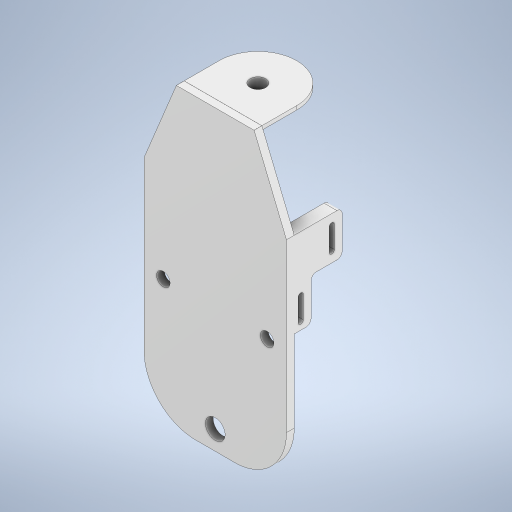
# Autodesk Inventor part: Electromagnet Gantry Plate
Saved by Autodesk Inventor 2023.2 (Build 272271030, 271C)
## iProperties
Created: 2023-04-10
Part Number: Electromagnet Gantry Plate
Material: PC/ABS Plastic
Document SubType Name: Modeling
Designer: ethan
Density: 0.357273 g/cm^3
Appearance: Smooth - White
Author: ethan
Autodesk Inventor part; units mm, degrees
ref_plane "YZ Plane" through (0, 0, 0) normal (1, 0, 0) x (0, 1, 0)
ref_plane "XZ Plane" through (0, 0, 0) normal (0, 1, 0) x (-1, 0, 0)
ref_plane "XY Plane" through (0, 0, 0) normal (0, 0, 1) x (1, 0, 0)
sketch "Sketch1" plane through (0, 0, 0) normal (0, 1, 0) x (-1, 0, 0)
  line L0 (0, 0) -> (55, 0)
  line L1 (55, 0) -> (55, -55)
  line L2 (55, -55) -> (0, -55)
  line L3 (0, -55) -> (0, 0)
  line L4 (47.55, -7.45) -> (7.45, -7.45) construction
  line L5 (7.45, -7.45) -> (7.45, -47.55) construction
  line L6 (7.45, -47.55) -> (47.55, -47.55) construction
  line L7 (47.55, -47.55) -> (47.55, -7.45) construction
  circle A0 centre (47.55, -7.45) radius 2.6
  circle A1 centre (47.55, -47.55) radius 2.6
  circle A2 centre (7.45, -47.55) radius 2.6
  circle A3 centre (7.45, -7.45) radius 2.6
  circle A4 centre (47.55, -7.45) radius 12.5 construction
  circle A5 centre (27.5, -7.45) radius 3.8
  line L8 (55, -55) -> (0, -55)
  line L9 (0, -55) -> (0, -139.9)
  line L10 (0, -139.9) -> (55, -139.9)
  line L11 (55, -139.9) -> (55, -55)
  point P0 (3.72, -55)
  dimension "d0" = 55
  dimension "d1" = 55
  dimension "d2" = 40.1
  dimension "d3" = 40.1
  dimension "d4" = 5.2
  dimension "d5" = 5.2
  dimension "d6" = 5.2
  dimension "d7" = 5.2
  dimension "d8" = 7.45
  dimension "d9" = 7.45
  dimension "d13" = 25
  dimension "d78" = 7.6
  dimension "d160" = 84.9
  constraints: 24 end point, 6 centre point, 6 parallel, 5 coincident, 3 horizontal, 3 perpendicular, 1 midpoint
  measures "d0" distance of L1.end L2.end
  measures "d1" distance of L0.end L1.end
  measures "d2" distance of L6.end L5.end
  measures "d3" distance of L5.end L4.end
  measures "d4" diameter of A0
  measures "d5" diameter of A3
  measures "d6" diameter of A1
  measures "d7" diameter of A2
  measures "d8" distance between parallel lines of L1 L7
  measures "d9" distance from line of L2 L5.end
  measures "d13" diameter of A4
  measures "d78" diameter of A5
  measures "d160" distance of L2.end L9.end
extrude "Extrusion1" add sketch "Sketch1" along normal blind 3 contours L0 L1 L2 L3 | L2 L11 L10 L9 | A0 | A3
fillet "Fillet1" radius 20 2 edges at (-55, 1.5, 0) (0, 1.5, 0)
ref_plane "Work Plane14" through (0, 0, 0) normal (0, 1, 0) x (1, 0, 0)
sketch "Sketch7" plane through (0, 0, 0) normal (0, 1, 0) x (1, 0, 0)
  line L0 (-19.45, 63) -> (-19.45, 55)
  line L1 (-35.55, 19.45) -> (-35.55, 63) projected
  line L2 (-19.45, 55) -> (-35.55, 55)
  line L3 (-35.55, 55) -> (-35.55, 63)
  line L4 (-35.55, 63) -> (-19.45, 63)
  line L5 (-19.45, 63) -> (-19.45, 55)
  circle A0 centre (-47.55, 47.55) radius 2.6 projected
  circle A1 centre (-47.55, 47.55) radius 12
  circle A2 centre (-7.45, 47.55) radius 2.6 projected
  circle A3 centre (-7.45, 47.55) radius 12
  point P0 (0, 0)
  point P1 (-53, 55)
  dimension "d67" = 24
  dimension "d68" = 24
  constraints: 10 end point, 2 centre point, 2 coincident, 2 parallel, 1 horizontal, 1 perpendicular
  measures "d67" diameter of A1
  measures "d68" diameter of A3
extrude "Extrusion9" add sketch "Sketch7" along normal blind 25 contours L0 L2 L1 L4
ref_plane "Work Plane2" through (-19.45, -5, -63) normal (0, 0, -1) x (-1, 0, 0)
sketch "Sketch9" plane through (-19.45, -5, -63) normal (0, 0, -1) x (-1, 0, 0)
  line L0 (0, 0) -> (0, 8) projected
  line L1 (16.1, 8) -> (16.1, 5) projected
  line L2 (0, 8) -> (16.1, 8)
  line L3 (4.55, 8) -> (11.55, 8) projected
  line L4 (8.05, 8) -> (8.05, 21.475)
  circle A0 centre (8.05, 21.475) radius 3
  point P0 (-19.45, 5)
  dimension "d54" = 13.475
  dimension "d55" = 6
  constraints: 4 end point, 1 centre point, 1 coincident, 1 midpoint, 1 perpendicular, 1 vertical
  measures "d54" distance of L4.start L4.end
  measures "d55" diameter of A0
extrude "Extrusion11" cut sketch "Sketch9" against normal through all
ref_plane "Work Plane12" through (-19.45, 0, -63) normal (0, 0, -1) x (-1, 0, 0)
sketch "Sketch10" plane through (-19.45, 0, -63) normal (0, 0, -1) x (-1, 0, 0)
  circle A0 centre (8.05, 16.475) radius 3 projected
  arc A1 (23.05, 16.475) -> (-6.95, 16.475) centre (8.05, 16.475) ccw
  line L0 (-6.95, 16.475) -> (-6.95, 0)
  line L1 (23.05, 16.475) -> (23.05, 0)
  line L2 (-6.95, 0) -> (23.05, 0)
  line L3 (33.55, 0) -> (-17.45, 0) projected
  point P0 (-19.45, 0)
  dimension "d60" = 30
  constraints: 6 end point, 2 point on circle, 2 tangent, 2 vertical, 1 centre point, 1 coincident, 1 collinear
  measures "d60" diameter of A1
extrude "Extrusion12" add sketch "Sketch10" against normal up to surface (8 mm away)
sketch "Sketch18" plane through (0, 3, 0) normal (0, 1, 0) x (1, 0, 0)
  circle A0 centre (-47.55, 47.55) radius 2.6 projected
  circle A1 centre (-47.55, 47.55) radius 12 construction
  line L0 (-47.55, 37.5) -> (0, 37.5)
  line L1 (0, 20) -> (0, 139.9) projected
  line L2 (-47.55, 54.5) -> (0, 54.5)
  line L3 (-47.55, 63) -> (0, 63)
  line L4 (-47.55, 72) -> (0, 72)
  line L5 (-47.55, 80.5) -> (0, 80.5)
  line L6 (-47.55, 139.9) -> (0, 139.9)
  point P0 (0, 0)
  point P1 (0, 63)
  point P2 (0, 83)
  dimension "d106" = 24
  dimension "d107" = 10.05
  dimension "d108" = 17
  dimension "d109" = 8.5
  dimension "d110" = 34.5
  dimension "d111" = 8.5
  dimension "d206" = 102.4
  constraints: 12 end point, 5 parallel, 1 centre point, 1 coincident, 1 horizontal, 1 point on line
  measures "d106" diameter of A1
  measures "d107" distance of A0.centre L0.start
  measures "d108" distance between parallel lines of L0 L2
  measures "d109" distance between parallel lines of L2 L3
  measures "d110" distance between parallel lines of L0 L4
  measures "d111" distance between parallel lines of L4 L5
  measures "d206" distance between parallel lines of L0 L6
sketch "Sketch27" plane through (-55, 0, -66.9) normal (-1, 0, 0) x (0, 0, 1)
  line L0 (-17.6, 21.5) -> (-17.6, 0)
  arc A0 (-5.1, 16.5) -> (-5.1, 18.5) centre (-5.1, 17.5) ccw
  line L1 (-13.6, 18.5) -> (-5.1, 18.5)
  line L2 (-5.1, 16.5) -> (-13.6, 16.5)
  arc A1 (-13.6, 18.5) -> (-13.6, 16.5) centre (-13.6, 17.5) ccw
  arc A2 (12.4, 4.5) -> (12.4, 6.5) centre (12.4, 5.5) ccw
  line L3 (3.9, 6.5) -> (12.4, 6.5)
  line L4 (12.4, 4.5) -> (3.9, 4.5)
  arc A3 (3.9, 6.5) -> (3.9, 4.5) centre (3.9, 5.5) ccw
  line L5 (0, 3) -> (0, 3) projected
  line L6 (-17.6, 0) -> (15.4, 0)
  line L7 (-73, 0) -> (46.9, 0) projected
  line L8 (15.4, 0) -> (15.4, 21.5)
  line L9 (15.4, 21.5) -> (-17.6, 21.5)
  line L10 (15.4, 9.5) -> (-1.1, 9.5)
  line L11 (-1.1, 9.5) -> (-1.1, 21.5)
  point P0 (66.9, 0)
  point P1 (-61, 3)
  point P2 (-14.6, 17.5)
  dimension "d164" = 1
  dimension "d165" = 1
  dimension "d166" = 1
  dimension "d167" = 1
  dimension "d172" = 5.5
  dimension "d173" = 17.5
  dimension "d182" = 8.5
  dimension "d183" = 8.5
  dimension "d185" = 2
  dimension "d187" = 3
  dimension "d188" = 3
  dimension "d189" = 3
  dimension "d191" = 54.5
  dimension "d192" = 3
  dimension "d194" = 3
  dimension "d195" = 2
  dimension "d196" = 17.5
  constraints: 20 end point, 9 point on circle, 4 centre point, 3 horizontal, 3 perpendicular, 2 parallel, 1 collinear, 1 horizontal alignment, 1 midpoint, 1 point on line, 1 vertical
  measures "d164" radius of A1
  measures "d165" radius of A0
  measures "d166" radius of A3
  measures "d167" radius of A2
  measures "d172" distance from line of L6 A2.centre
  measures "d173" distance from line of L6 A0.centre
  measures "d182" distance of A2.centre A3.centre
  measures "d183" distance of A0.centre A1.centre
  measures "d185" distance between parallel lines of L3 L4
  measures "d187" distance from line of L8 A2.centre
  measures "d188" distance between parallel lines of L9 L1
  measures "d189" distance between parallel lines of L10 L3
  measures "d191" horizontal distance of point (66.9, 0) A2.centre
  measures "d192" distance edge to line of A0 L11
  measures "d194" distance from line of point (-14.6, 17.5) L0
  measures "d195" distance between parallel lines of L1 L2
  measures "d196" horizontal distance of A0.centre A2.centre
extrude "Extrusion29" add sketch "Sketch27" against normal blind 5 contours L9 L11 L10 L8 L6 L0
fillet "Fillet13" radius 2 3 edges at (-52.5, 9.5, -51.5) (-52.5, 21.5, -68) (-52.5, 21.5, -84.5)
ref_plane "Work Plane10" through (-27.5, 0, -20) normal (-1, 0, 0) x (0, 0, 1)
mirror "Mirror6" about plane through (-27.5, 0, -20) normal (-1, 0, 0) of "Extrusion29", "Fillet13"
chamfer "Chamfer5" distance 6.5 angle 45 3 edges at (-27.5, 31.475, -55) (-42.5, 9.7375, -55) (-12.5, 9.7375, -55)
chamfer "Chamfer6" distance 6 angle 45 1 edges at (-27.5, 3, -55)
ref_plane "Work Plane16" through (0, 0, -114.9) normal (0, 0, -1) x (-1, 0, 0)
move faces "Move1" translate (0, 0, -51.9) faces at (-27.6205, 6.499, -63) (-12.6942, 18.8812, -62.5) (-42.5, 7.4917, -62.5) (-40.3333, 9.4917, -59.3333) (-39.1188, 18.2262, -58.25) (-14.6667, 9.4917, -59.3333) (-12.5, 7.4917, -62) (-27.6205, 10.499, -55) (-28.3333, 7, -53) (-30.4903, 16.2336, -57.6667)
sketch "Sketch29" plane through (0, 3, 0) normal (0, 1, 0) x (1, 0, 0)
  line L0 (0, 139.9) -> (-55, 139.9) projected
  line L1 (0, 20) -> (0, 139.9) projected
  line L2 (-55, 139.9) -> (0, 139.9)
  line L3 (0, 139.9) -> (0, 114.877)
  line L4 (0, 114.877) -> (-55, 114.877)
  line L5 (-55, 114.877) -> (-55, 139.9)
  line L6 (-42.5, 114.9) -> (-42.5, 113.4) projected
  line L7 (-50, 84.5) -> (-55, 84.5) projected
  line L8 (-42.5, 114.9) -> (-55, 84.5)
  line L9 (-55, 84.5) -> (-55, 114.877)
  line L10 (-12.5, 114.9) -> (-12.5, 113.4) projected
  line L11 (-12.5, 114.9) -> (0, 84.5)
  line L12 (0, 84.5) -> (0, 114.877)
  line L13 (0, 84.5) -> (0, 139.9) projected
  point P0 (0, 0)
  point P1 (-42.5, 114.877)
  point P2 (-12.5, 114.877)
  constraints: 16 end point, 2 parallel, 2 perpendicular, 1 collinear, 1 horizontal, 1 point on line
extrude "Extrusion31" cut sketch "Sketch29" against normal through all contours L1 L4 L11 L10 L6 L8 L5 L0 | L1 L11 L4 | L4 L8 L9
fillet "Fillet14" radius 2 2 edges at (-52.5, 9.5, -68) (-2.5, 9.5, -68)
equation "\"d1\" = d0"
equation "\"d3\" = d2"
equation "\"d5\" = d4"
equation "\"d6\" = d4"
equation "\"d7\" = d4"
equation "\"d8\" = -0.5 * d2 + 0.5 * d0"
equation "\"d9\" = -0.5 * d3 + 0.5 * d1"
body "Solid1"
